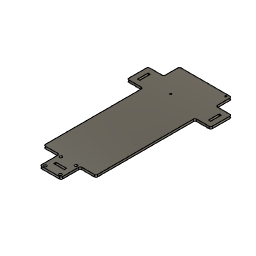
Main Body (Autodesk Fusion 360 design; units mm, degrees)
Autodesk Fusion 360 part; units mm, degrees
sketch "Sketch1" plane through (0, 0, 0) normal (0, 0, 1) x (1, 0, 0)
  line L0 (50, -130) -> (-50, -130)
  line L1 (-80, -100) -> (-80, -60)
  line L2 (80, -60) -> (80, -100)
  line L3 (-20, 130) -> (-20, 167)
  line L4 (-20, 167) -> (20, 167)
  line L5 (20, 167) -> (20, 130)
  circle A0 centre (14.5, 132.5) radius 2.5
  circle A1 centre (14.5, 162.5) radius 2.5
  line L6 (0, 180) -> (0, -175) construction
  line L7 (-50, 130) -> (-20, 130)
  line L8 (20, 130) -> (50, 130)
  circle A2 centre (-14.5, 162.5) radius 2.5
  circle A3 centre (-14.5, 132.5) radius 2.5
  line L9 (-80, -60) -> (-50, -60)
  line L10 (50, -60) -> (80, -60)
  line L11 (80, -100) -> (50, -100)
  line L12 (-50, -100) -> (-80, -100)
  line L13 (50, 130) -> (50, -60)
  line L14 (50, -100) -> (50, -130)
  line L15 (-50, -130) -> (-50, -100)
  line L16 (-50, -60) -> (-50, 130)
  line L17 (10, 150.5) -> (-10, 150.5)
  line L18 (-10, 150.5) -> (-10, 146.5)
  line L19 (-10, 146.5) -> (10, 146.5)
  line L20 (10, 146.5) -> (10, 150.5)
  line L21 (70, -90) -> (66, -90)
  line L22 (66, -90) -> (66, -70)
  line L23 (66, -70) -> (70, -70)
  line L24 (70, -70) -> (70, -90)
  line L25 (-70, -70) -> (-70, -90)
  line L26 (-66, -90) -> (-66, -70)
  line L27 (-66, -70) -> (-70, -70)
  line L28 (-70, -90) -> (-66, -90)
  circle A4 centre (-43, -126) radius 1.5
  circle A5 centre (13.5, -77) radius 1.5
  point P0 (0, -80)
  point P1 (0, 148.5)
  point P2 (0, 148.5)
  point P3 (68, -80)
  dimension "d1" = 100
  dimension "d3" = 160
  dimension "d4" = 40
  dimension "d5" = 30
  dimension "d6" = 30
  dimension "d7" = 40
  dimension "d8" = 37
  dimension "d10" = 18.5
  dimension "d14" = 5
  dimension "d15" = 20
  dimension "d16" = 4
  dimension "d18" = 4
  dimension "d19" = 20
  dimension "d20" = 10
  dimension "d21" = 20
  dimension "d24" = 3
  dimension "d27" = 3
  dimension "d28" = 53
  dimension "d29" = 4
  dimension "d30" = 7
  dimension "d31" = 56.5
  dimension "d34" = 297
  dimension "d39" = 4.5
  dimension "d40" = 5.5
  dimension "d41" = 30
  dimension "d42" = 12
  constraint horizontal L0
  constraint perpendicular L0 L15
  constraint parallel L0 L7
  constraint parallel L13 L15
  constraint horizontal L11
  constraint perpendicular L1 L11
  constraint parallel L9 L11
  constraint parallel L1 L2
  constraint parallel L3 L5
  constraint collinear L7 L8
  constraint symmetric A0 L6 A3
  constraint symmetric A1 L6 A2
  constraint collinear L9 L10
  constraint coincident L9.end L15
  constraint collinear L11 L12
  constraint coincident L11.end L13
  constraint collinear L13 L14
  constraint collinear L15 L16
  constraint horizontal L17
  constraint perpendicular L17 L18
  constraint parallel L17 L19
  constraint parallel L18 L20
  constraint coincident P2 P1
  constraint horizontal L21
  constraint perpendicular L21 L22
  constraint parallel L21 L23
  constraint parallel L22 L24
  constraint symmetric L6 L21.start L25.end
  constraint symmetric L6 L21.end L26.start
  constraint symmetric L6 L22.end L26.end
  constraint symmetric L6 L23.end L25.start
  measures "d1" distance of L7.start L8.end
  measures "d3" distance of L1.end L2.start
  measures "d4" distance of L1.start L1.end
  measures "d5" distance of L0 L11
  measures "d6" distance of L2 L13
  measures "d7" distance of L3.end L4.end
  measures "d8" distance of L3.start L3.end
  measures "d10" distance of P2 L7
  measures "d14" diameter of A1
  measures "d15" distance of L18.end L19.end
  measures "d16" distance of L17.end L18.end
  measures "d18" distance of L22.end L23.end
  measures "d19" distance of L21.end L22.end
  measures "d20" distance of L2 L24
  measures "d21" distance of L11 P3
  measures "d24" diameter of A4
  measures "d27" diameter of A5
  measures "d28" distance of L0 A5.centre
  measures "d29" distance of L0 A4.centre
  measures "d30" distance of L15 A4.centre
  measures "d31" horizontal distance of A4.centre A5.centre
  measures "d34" distance of L0 L4
  measures "d39" distance of L4 A1.centre
  measures "d40" distance of L5 A1.centre
  measures "d41" distance of A0.centre A1.centre
  measures "d42" distance of A1.centre L17
extrude "Extrude1" add sketch "Sketch1" along normal blind 4
fillet "Fillet1" radius 3 2 edges at (20, 167, 2) (-20, 167, 2)
fillet "Fillet2" radius 3 14 edges at (-20, 130, 2) (-50, 130, 2) (20, 130, 2) (50, 130, 2) (50, -60, 2) (80, -60, 2) (80, -100, 2) (50, -100, 2) (50, -130, 2) (-50, -130, 2) (-50, -100, 2) (-80, -100, 2) (-80, -60, 2) (-50, -60, 2)
move_body "Move1" bodies 1 to x (-1, 0, 0) y (0, -1, 0) z (0, 0, 1) at (-160, -260, 0)
